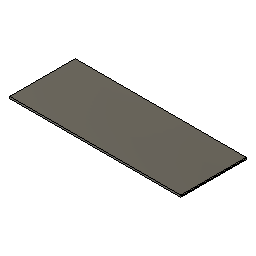
duct_panel (Autodesk Fusion 360 design; units mm, degrees)
part number: 2026-08-26-07-13-40-754
Autodesk Fusion 360 part; units mm, degrees
sketch "Panel outline" plane through (0, 0, 0) normal (0, 0, 1) x (1, 0, 0)
  line L0 (-97.22, 0) -> (97.22, 0)
  line L1 (97.22, 0) -> (97.22, 74)
  line L2 (97.22, 74) -> (-97.22, 74)
  line L3 (-97.22, 74) -> (-97.22, 0)
extrude "Panel" add sketch "Panel outline" along normal blind 2.2
chamfer "Groove lead-in" distance 0.6 angle 45 4 edges at (97.22, 37, 0) (97.22, 37, 2.2) (-97.22, 37, 0) (-97.22, 37, 2.2)
named bodies: "Duct Panel"
